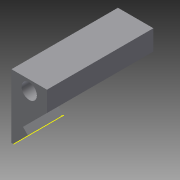
# Autodesk Inventor part: recessedCoverslip_v1
Saved by Autodesk Inventor 2013 (Build 170138000, 138)
## iProperties
Created: 2014-12-18
Part Number: recessedCoverslip_v1
Material: Generic
Document SubType Name: Modeling
Designer: 120pa
Density: 1 g/cm^3
Author: 120pa
Autodesk Inventor part; units mm, degrees
ref_plane "YZ Plane" through (0, 0, 0) normal (1, 0, 0) x (0, 1, 0)
ref_plane "XZ Plane" through (0, 0, 0) normal (0, 1, 0) x (-1, 0, 0)
ref_plane "XY Plane" through (0, 0, 0) normal (0, 0, 1) x (1, 0, 0)
sketch "Sketch1" plane through (0, 0, 0) normal (0, 1, 0) x (-1, 0, 0)
  line L0 (0, -5.6886) -> (6.7556, -12.4442)
  line L1 (6.7556, -12.4442) -> (5.3414, -13.8584)
  line L2 (9.5, -18.017) -> (5.3414, -13.8584)
  line L3 (10, -18.017) -> (9.5, -18.017)
  line L4 (10, -18.017) -> (10, 0)
  line L5 (0, 0) -> (10, 0)
  line L6 (0, 0) -> (0, -5.6886)
  circle A0 centre (5, -2.8443) radius 1.339
  constraints: 14 end point, 1 centre point
extrude "Extrusion1" add sketch "Sketch1" along normal blind 10
sketch "Sketch2" plane through (0, 10, 0) normal (0, 1, 0) x (1, 0, 0)
  line L0 (0, 5.6886) -> (-10, 5.6886)
  line L1 (-10, 5.6886) -> (-10, 0)
  line L2 (-10, 0) -> (0, 0)
  line L3 (0, 0) -> (0, 5.6886)
  constraints: 8 end point
extrude "Extrusion2" add sketch "Sketch2" along normal blind 20
sketch "Sketch3" plane through (0, 0, 0) normal (0, -1, 0) x (1, 0, 0)
  circle A0 centre (-5, -2.8443) radius 1.339 projected
hole "Hole1" at (-5, 0, -2.8443) direction (0, 1, 0) diameter 4.318 depth 31 tip angle 118
sketch "Sketch4" plane through (-9.5, 0, -18.017) normal (0.7071, 0, -0.7071) x (-0.7071, 0, -0.7071)
  circle A0 centre (-2.9406, 5) radius 2.55
  point P0 (-19.4575, 0)
  dimension "d11" = 5.1
  constraints: 1 centre point
  measures "d11" diameter of A0
extrude "Extrusion3" cut sketch "Sketch4" against normal blind 0.1
sketch "Sketch5" plane through (-7.4914, 5, -15.867) normal (0.7071, 0, -0.7071) x (-0.7071, 0, -0.7071)
  circle A0 centre (0, 0) radius 2
  point P0 (-16.5169, -5)
  dimension "d15" = 4
  constraints: 1 centre point
  measures "d15" diameter of A0
extrude "Extrusion4" cut sketch "Sketch5" against normal blind 10
sketch "Sketch6" plane through (-9.5, 0, -18.017) normal (0.7071, 0, -0.7071) x (-0.7071, 0, -0.7071)
  circle A0 centre (-2.9406, 5) radius 2.55 projected
  line L0 (-5.8811, 0) -> (0, 0) projected
  line L1 (0, 0) -> (0, 10) projected
  line L2 (-5.8811, 10) -> (0, 10) projected
  line L3 (-5.8811, 0) -> (-5.8811, 10) projected
  point P0 (-19.4575, 0)
hole "Hole2" at (-7.3787, 1.3, -15.8957) direction (-0.7071, 0, 0.7071) diameter 1.778 depth 8 tip angle 118 clearance for "Flat Head Machine Screw (82)" size "#0" standard "Ansi Unified Screw Threads"
hole "Hole3" at (-7.3787, 8.7, -15.8957) direction (-0.7071, 0, 0.7071) diameter 1.778 depth 8 tip angle 118 clearance for "Flat Head Machine Screw (82)" size "#0" standard "Ansi Unified Screw Threads"
body "Solid1"
